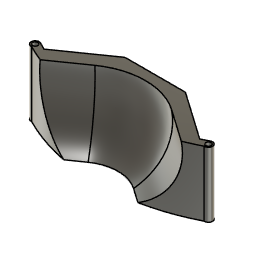
ボール壁　ピッタリ２ v1 (Autodesk Fusion 360 design; units mm, degrees)
Autodesk Fusion 360 part; units mm, degrees
sketch "スケッチ1" plane through (0, 0, 0) normal (0, 0, 1) x (1, 0, 0)
  line L0 (0, 0) -> (-103.75, 0) construction
  line L1 (41.3768, 78.5707) -> (78.5707, 41.3768)
  arc A0 (41.3768, -78.5707) -> (41.3768, -81.3991) centre (42.7911, -79.9849) ccw
  line L2 (-78.5707, 41.3768) -> (-41.3768, 78.5707)
  line L3 (78.5707, -41.3768) -> (41.3768, -78.5707)
  arc A1 (41.3768, 81.3991) -> (41.3768, 78.5707) centre (42.7911, 79.9849) ccw
  circle A2 centre (-47.3873, -90.2379) radius 2.215
  circle A3 centre (-90.2379, 47.3873) radius 2.215
  line L4 (-50.5692, -90.5915) -> (-41.3768, -81.3991)
  circle A4 centre (-47.3873, 90.2379) radius 1.465
  circle A5 centre (-90.2379, 47.3873) radius 1.465
  circle A6 centre (90.2379, -47.3873) radius 1.465
  line L5 (90.5915, 50.5692) -> (81.3991, 41.3768)
  line L6 (-90.5915, 50.5692) -> (-81.3991, 41.3768)
  circle A7 centre (-90.2379, -47.3873) radius 2.215
  circle A8 centre (90.2379, 47.3873) radius 1.465
  line L7 (100, 0) -> (95.4059, 0)
  circle A9 centre (47.3873, -90.2379) radius 1.465
  arc A10 (-41.3768, 78.5707) -> (-41.3768, 81.3991) centre (-42.7911, 79.9849) ccw
  circle A11 centre (47.3873, 90.2379) radius 2.215
  circle A12 centre (-90.2379, -47.3873) radius 1.465
  line L8 (-50.5692, 90.5915) -> (-41.3768, 81.3991)
  line L9 (50.5692, -90.5915) -> (41.3768, -81.3991)
  circle A13 centre (47.3873, 90.2379) radius 1.465
  circle A14 centre (-47.3873, 90.2379) radius 2.215
  line L10 (-90.5915, -50.5692) -> (-81.3991, -41.3768)
  arc A15 (-81.3991, 41.3768) -> (-78.5707, 41.3768) centre (-79.9849, 42.7911) ccw
  line L11 (50.5692, -90.5915) -> (48.8015, -88.8237)
  circle A16 centre (-47.3873, -90.2379) radius 1.465
  circle A17 centre (0, 0) radius 99.75
  circle A18 centre (0, 0) radius 103.75
  circle A19 centre (90.2379, 47.3873) radius 2.215
  arc A20 (-78.5707, -41.3768) -> (-81.3991, -41.3768) centre (-79.9849, -42.7911) ccw
  arc A21 (78.5707, 41.3768) -> (81.3991, 41.3768) centre (79.9849, 42.7911) ccw
  circle A22 centre (90.2379, -47.3873) radius 2.215
  line L12 (50.5692, 90.5915) -> (41.3768, 81.3991)
  circle A23 centre (47.3873, -90.2379) radius 2.215
  arc A24 (-41.3768, -81.3991) -> (-41.3768, -78.5707) centre (-42.7911, -79.9849) ccw
  line L13 (0, 0) -> (-103.75, 0) construction
  line L14 (90.5915, -50.5692) -> (81.3991, -41.3768)
  arc A25 (81.3991, -41.3768) -> (78.5707, -41.3768) centre (79.9849, -42.7911) ccw
  line L15 (-41.3768, -78.5707) -> (-78.5707, -41.3768)
  line L16 (0, 0) -> (-103.75, 0) construction
  line L17 (41.3768, 78.5707) -> (78.5707, 41.3768)
  arc A26 (41.3768, -78.5707) -> (41.3768, -81.3991) centre (42.7911, -79.9849) ccw
  line L18 (-78.5707, 41.3768) -> (-41.3768, 78.5707)
  line L19 (78.5707, -41.3768) -> (41.3768, -78.5707)
  arc A27 (41.3768, 81.3991) -> (41.3768, 78.5707) centre (42.7911, 79.9849) ccw
  circle A28 centre (-47.3873, -90.2379) radius 2.215
  circle A29 centre (-90.2379, 47.3873) radius 2.215
  line L20 (-50.5692, -90.5915) -> (-41.3768, -81.3991)
  circle A30 centre (-47.3873, 90.2379) radius 1.465
  circle A31 centre (-90.2379, 47.3873) radius 1.465
  circle A32 centre (90.2379, -47.3873) radius 1.465
  line L21 (90.5915, 50.5692) -> (81.3991, 41.3768)
  line L22 (-90.5915, 50.5692) -> (-81.3991, 41.3768)
  circle A33 centre (-90.2379, -47.3873) radius 2.215
  circle A34 centre (90.2379, 47.3873) radius 1.465
  line L23 (100, 0) -> (95.4059, 0)
  circle A35 centre (47.3873, -90.2379) radius 1.465
  arc A36 (-41.3768, 78.5707) -> (-41.3768, 81.3991) centre (-42.7911, 79.9849) ccw
  circle A37 centre (47.3873, 90.2379) radius 2.215
  circle A38 centre (-90.2379, -47.3873) radius 1.465
  line L24 (-50.5692, 90.5915) -> (-41.3768, 81.3991)
  line L25 (50.5692, -90.5915) -> (41.3768, -81.3991)
  circle A39 centre (47.3873, 90.2379) radius 1.465
  circle A40 centre (-47.3873, 90.2379) radius 2.215
  line L26 (-90.5915, -50.5692) -> (-81.3991, -41.3768)
  arc A41 (-81.3991, 41.3768) -> (-78.5707, 41.3768) centre (-79.9849, 42.7911) ccw
  line L27 (50.5692, -90.5915) -> (48.8015, -88.8237)
  circle A42 centre (-47.3873, -90.2379) radius 1.465
  circle A43 centre (0, 0) radius 99.75
  circle A44 centre (0, 0) radius 103.75
  circle A45 centre (90.2379, 47.3873) radius 2.215
  arc A46 (-78.5707, -41.3768) -> (-81.3991, -41.3768) centre (-79.9849, -42.7911) ccw
  arc A47 (78.5707, 41.3768) -> (81.3991, 41.3768) centre (79.9849, 42.7911) ccw
  circle A48 centre (90.2379, -47.3873) radius 2.215
  line L28 (50.5692, 90.5915) -> (41.3768, 81.3991)
  circle A49 centre (47.3873, -90.2379) radius 2.215
  arc A50 (-41.3768, -81.3991) -> (-41.3768, -78.5707) centre (-42.7911, -79.9849) ccw
  line L29 (0, 0) -> (-103.75, 0) construction
  line L30 (90.5915, -50.5692) -> (81.3991, -41.3768)
  arc A51 (81.3991, -41.3768) -> (78.5707, -41.3768) centre (79.9849, -42.7911) ccw
  line L31 (-41.3768, -78.5707) -> (-78.5707, -41.3768)
  line L32 (-42.545, -90.2219) -> (-16.4968, -72)
  line L33 (-16.4968, -72) -> (0, -72)
  line L34 (16.4968, -72) -> (0, -72)
  line L35 (42.545, -90.2219) -> (16.4968, -72)
  dimension "d2" = 360
  dimension "d3" = 13
  dimension "d4" = 2
  dimension "d5" = 2
  dimension "d7" = 360
  dimension "d8" = 13
  dimension "d9" = 2
  dimension "d10" = 2
  constraint coincident L0.start A17.centre
  constraint coincident L4.start A18
  constraint tangent A20 L15
  constraint parallel L9 L11
  constraint concentric A9 A23
  constraint coincident L4.start A44
  constraint tangent A46 L31
  constraint parallel L25 L27
  constraint concentric A35 A49
  constraint coincident A17 L32.start
  measures "d3" distance of L4.end L4.start
  measures "d4" distance of L4.end A24.centre
  measures "d5" distance of A24.end A24.centre
  measures "d8" distance of L4.end L4.start
  measures "d9" distance of L4.end A24.centre
  measures "d10" distance of A24.end A24.centre
extrude "押し出し1" add sketch "スケッチ1" along normal blind 35.5 contours L9 L11 A23 L25 L27 A49 | L9 L11 A17 A18 A23 L25 L27 A43 A44 A49 | A17 A23 A43 A49 | A2 A17 A18 A23 A28 A43 A44 A49 | A18 A23 A44 A49 | A17 A43 L32 L33 L34 L35 | A2 L4 A17 A18 A28 L20 A43 A44 | A2 A18 A28 A44 | A2 A17 A28 A43 | A2 L4 A28 L20
ref_plane "作業平面1" through (0, 0, 30) normal (0, 0, 1) x (1, 0, 0)
sketch "スケッチ2" plane through (0, 0, 30) normal (0, 0, 1) x (1, 0, 0)
  arc A0 (37, -114) -> (-37, -114) centre (0, -114) ccw
  circle A1 centre (-90.2379, 47.3873) radius 1.465
  circle A2 centre (0, 0) radius 99.75
  arc A3 (-81.3991, 41.3768) -> (-78.5707, 41.3768) centre (-79.9849, 42.7911) ccw
  arc A4 (-41.3768, 78.5707) -> (-41.3768, 81.3991) centre (-42.7911, 79.9849) ccw
  circle A5 centre (-47.3873, 90.2379) radius 1.465
  circle A6 centre (-90.2379, 47.3873) radius 2.215
  line L0 (78.5707, -41.3768) -> (41.3768, -78.5707)
  arc A7 (81.3991, -41.3768) -> (78.5707, -41.3768) centre (79.9849, -42.7911) ccw
  line L1 (50.5692, -90.5915) -> (41.3768, -81.3991)
  circle A8 centre (90.2379, -47.3873) radius 1.465
  arc A9 (81.3991, -41.3768) -> (78.5707, -41.3768) centre (79.9849, -42.7911) ccw
  circle A10 centre (-90.2379, -47.3873) radius 1.465
  circle A11 centre (-90.2379, -47.3873) radius 2.215
  circle A12 centre (-47.3873, -90.2379) radius 1.465
  circle A13 centre (47.3873, -90.2379) radius 2.215
  line L2 (50.5692, -90.5915) -> (48.8015, -88.8237)
  line L3 (50.5692, -90.5915) -> (41.3768, -81.3991)
  arc A14 (-41.3768, -81.3991) -> (-41.3768, -78.5707) centre (-42.7911, -79.9849) ccw
  line L4 (-90.5915, -50.5692) -> (-81.3991, -41.3768)
  circle A15 centre (90.2379, -47.3873) radius 1.465
  circle A16 centre (90.2379, -47.3873) radius 2.215
  arc A17 (41.3768, -78.5707) -> (41.3768, -81.3991) centre (42.7911, -79.9849) ccw
  arc A18 (-41.3768, -81.3991) -> (-41.3768, -78.5707) centre (-42.7911, -79.9849) ccw
  line L5 (-50.5692, -90.5915) -> (-41.3768, -81.3991)
  circle A19 centre (-47.3873, -90.2379) radius 1.465
  arc A20 (41.3768, 81.3991) -> (41.3768, 78.5707) centre (42.7911, 79.9849) ccw
  circle A21 centre (90.2379, -47.3873) radius 2.215
  circle A22 centre (47.3873, 90.2379) radius 1.465
  line L6 (90.5915, -50.5692) -> (81.3991, -41.3768)
  line L7 (50.5692, 90.5915) -> (41.3768, 81.3991)
  arc A23 (78.5707, 41.3768) -> (81.3991, 41.3768) centre (79.9849, 42.7911) ccw
  circle A24 centre (-90.2379, -47.3873) radius 1.465
  arc A25 (-78.5707, -41.3768) -> (-81.3991, -41.3768) centre (-79.9849, -42.7911) ccw
  line L8 (50.5692, -90.5915) -> (48.8015, -88.8237)
  line L9 (90.5915, 50.5692) -> (81.3991, 41.3768)
  circle A26 centre (47.3873, 90.2379) radius 2.215
  arc A27 (-78.5707, -41.3768) -> (-81.3991, -41.3768) centre (-79.9849, -42.7911) ccw
  line L10 (-41.3768, -78.5707) -> (-78.5707, -41.3768)
  arc A28 (41.3768, 81.3991) -> (41.3768, 78.5707) centre (42.7911, 79.9849) ccw
  circle A29 centre (47.3873, -90.2379) radius 1.465
  line L11 (-90.5915, -50.5692) -> (-81.3991, -41.3768)
  line L12 (90.5915, 50.5692) -> (81.3991, 41.3768)
  line L13 (41.3768, 78.5707) -> (78.5707, 41.3768)
  line L14 (-16.4968, -72) -> (0, -72)
  line L15 (42.545, -90.2219) -> (16.4968, -72)
  circle A30 centre (47.3873, -90.2379) radius 2.215
  line L16 (100, 0) -> (95.4059, 0)
  circle A31 centre (-90.2379, -47.3873) radius 2.215
  line L17 (90.5915, -50.5692) -> (81.3991, -41.3768)
  circle A32 centre (90.2379, 47.3873) radius 1.465
  line L18 (-42.545, -90.2219) -> (-16.4968, -72)
  arc A33 (41.3768, -78.5707) -> (41.3768, -81.3991) centre (42.7911, -79.9849) ccw
  line L19 (-50.5692, -90.5915) -> (-41.3768, -81.3991)
  circle A34 centre (90.2379, 47.3873) radius 2.215
  line L20 (-41.3768, -78.5707) -> (-78.5707, -41.3768)
  circle A35 centre (47.3873, -90.2379) radius 1.465
  circle A36 centre (47.3873, 90.2379) radius 2.215
  circle A37 centre (90.2379, 47.3873) radius 1.465
  circle A38 centre (-47.3873, -90.2379) radius 2.215
  circle A39 centre (-47.3873, -90.2379) radius 2.215
  line L21 (50.5692, 90.5915) -> (41.3768, 81.3991)
  line L22 (16.4968, -72) -> (0, -72)
  line L23 (100, 0) -> (95.4059, 0)
  line L24 (78.5707, -41.3768) -> (41.3768, -78.5707)
  line L25 (0, 0) -> (-103.75, 0) construction
  line L26 (-90.5915, 50.5692) -> (-81.3991, 41.3768)
  line L27 (-50.5692, 90.5915) -> (-41.3768, 81.3991)
  line L28 (0, 0) -> (-103.75, 0) construction
  line L29 (-78.5707, 41.3768) -> (-41.3768, 78.5707)
  line L30 (0, 0) -> (-103.75, 0) construction
  line L31 (-78.5707, 41.3768) -> (-41.3768, 78.5707)
  circle A40 centre (-47.3873, 90.2379) radius 1.465
  circle A41 centre (-90.2379, 47.3873) radius 1.465
  line L32 (-50.5692, 90.5915) -> (-41.3768, 81.3991)
  circle A42 centre (-47.3873, 90.2379) radius 2.215
  circle A43 centre (0, 0) radius 103.75
  circle A44 centre (-47.3873, 90.2379) radius 2.215
  line L33 (0, 0) -> (-103.75, 0) construction
  circle A45 centre (0, 0) radius 103.75
  line L34 (-90.5915, 50.5692) -> (-81.3991, 41.3768)
  circle A46 centre (0, 0) radius 99.75
  arc A47 (78.5707, 41.3768) -> (81.3991, 41.3768) centre (79.9849, 42.7911) ccw
  circle A48 centre (47.3873, 90.2379) radius 1.465
  line L35 (41.3768, 78.5707) -> (78.5707, 41.3768)
  circle A49 centre (90.2379, 47.3873) radius 2.215
  arc A50 (-41.3768, 78.5707) -> (-41.3768, 81.3991) centre (-42.7911, 79.9849) ccw
  arc A51 (-81.3991, 41.3768) -> (-78.5707, 41.3768) centre (-79.9849, 42.7911) ccw
  circle A52 centre (-90.2379, 47.3873) radius 2.215
  line L36 (39.0123, -96.1359) -> (4.51, -72)
  line L37 (-39.0123, -96.1359) -> (-4.51, -72)
  line L38 (-37, -114) -> (37, -114)
  dimension "d15" = 360
  dimension "d17" = 360
  dimension "d18" = 13
  dimension "d19" = 2
  dimension "d20" = 2
  dimension "d21" = 13
  dimension "d22" = 2
  dimension "d23" = 2
  constraint coincident A2.centre L25.start
  constraint coincident L5.start A43
  constraint tangent A27 L20
  constraint parallel L1 L2
  constraint concentric A30 A35
  constraint coincident L5.start A45
  constraint tangent A25 L10
  constraint parallel L3 L8
  constraint concentric A13 A29
  constraint coincident L18.start A46
  constraint coincident A43 L36.start
  constraint coincident L22 L36.end
  constraint horizontal L38
  measures "d18" distance of L5.start A14.start
  measures "d19" distance of A14.centre A14.start
  measures "d20" distance of A14.centre A14.end
  measures "d21" distance of A14.start L5.start
  measures "d22" distance of A14.start A14.centre
  measures "d23" distance of A14.end A14.centre
revolve "回転1" cut sketch "スケッチ2" angle 360 about axis through (-37, -114, 30) along (1, 0, 0) contours A0 A43 A45 L38 | A0 A2 A43 A45 A46 | A0 A2 A46
ref_plane "作業平面2" through (0, 0, 30) normal (0, 0, 1) x (1, 0, 0)
sketch "スケッチ3" plane through (0, 0, 30) normal (0, 0, 1) x (1, 0, 0)
  arc A0 (37, -114) -> (-37, -114) centre (0, -114) ccw
  line L0 (39.0123, -96.1359) -> (4.51, -72)
  line L1 (-39.0123, -96.1359) -> (-4.51, -72)
  line L2 (0, -114) -> (21.209, -83.6817)
  line L3 (0, -114) -> (41.1821, -142.8087)
  line L4 (41.1821, -142.8087) -> (39.0123, -96.1359)
  constraint coincident A0.centre L2.start
  constraint coincident L0 L2.end
  constraint perpendicular L0 L2
  constraint perpendicular L2 L3
revolve "回転2" cut sketch "スケッチ3" angle 360 about axis through (0, -114, 30) along (0.819407, -0.573212, 0)
ref_plane "作業平面3" through (0, 0, 30) normal (0, 0, 1) x (1, 0, 0)
sketch "スケッチ4" plane through (0, 0, 30) normal (0, 0, 1) x (1, 0, 0)
  line L0 (0, -114) -> (21.209, -83.6817)
  line L1 (0, -114) -> (41.1821, -142.8087)
  line L2 (41.1821, -142.8087) -> (39.0123, -96.1359)
  line L3 (39.0123, -96.1359) -> (4.51, -72)
  line L4 (0, -100) -> (0, -125)
  line L5 (0, -114) -> (-21.209, -83.6817)
  line L6 (-39.0123, -96.1359) -> (-4.51, -72)
  line L7 (-41.1821, -142.8087) -> (-39.0123, -96.1359)
  line L8 (0, -114) -> (-41.1821, -142.8087)
  constraint coincident L0.end L3
  constraint perpendicular L0 L3
  constraint perpendicular L0 L1
  constraint vertical L4
  constraint symmetric L3.end L4 L6.end
  constraint symmetric L2.end L4 L6.start
  constraint symmetric L0.end L4 L5.end
  constraint symmetric L0.start L4 L1.start
  constraint symmetric L1.end L4 L7.start
revolve "回転3" cut sketch "スケッチ4" angle 360 about axis through (0, -114, 30) along (-0.819407, -0.573212, 0) contours L5 L6 L7 L8
